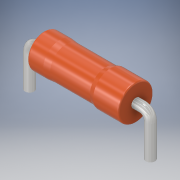
# Autodesk Inventor part: Res
Saved by Autodesk Inventor 2017 (Build 210142000, 142)
## iProperties
Created: 2016-07-07
Part Number: Res
Material: Generic
Document SubType Name: Modeling
Designer: Home
Density: 1 g/cm^3
Appearance: Default
Author: Home
Autodesk Inventor part; units mm, degrees
sketch "Sketch4" plane through (0, 0, 0) normal (0, 1, 0) x (-1, 0, 0)
  circle A0 centre (3.81, 0) radius 0.29
  circle A1 centre (-3.81, 0) radius 0.29
  point P0 (0, 0)
  dimension "d24" = 3.81
  dimension "d25" = 3.81
  dimension "d26" = 0.58
  dimension "d27" = 0.58
  constraints: 2 centre point
  measures "d24" distance of point (0, 0) A0.centre
  measures "d25" distance of A1.centre point (0, 0)
  measures "d26" diameter of A0
  measures "d27" diameter of A1
extrude "Extrusion2" add sketch "Sketch4" along normal blind 1.1 and the other way blind 1
sketch "Cable-Outline" plane through (0, 0, 0) normal (0, 0, 1) x (1, 0, 0)
  arc A0 (-3.32, 1.88) -> (-4.1, 1.1) centre (-3.32, 1.1) ccw construction
  line L0 (-3.52, 1.1) -> (-4.1, 1.1) construction
  arc A1 (-3.32, 1.3) -> (-3.52, 1.1) centre (-3.32, 1.1) ccw construction
  line L1 (4.1, 1.1) -> (3.52, 1.1) construction
  arc A2 (3.52, 1.1) -> (3.32, 1.3) centre (3.32, 1.1) ccw construction
  arc A3 (4.1, 1.1) -> (3.32, 1.88) centre (3.32, 1.1) ccw construction
  line L2 (3.32, 1.1) -> (3.32, 1.88) construction
  line L3 (3.32, 1.1) -> (4.1, 1.1) construction
  line L4 (-3.32, 1.88) -> (3.32, 1.88) construction
  line L5 (-3.32, 1.3) -> (3.32, 1.3) construction
  line L6 (-3.4614, 1.2414) -> (-3.8715, 1.6515) construction
  line L7 (3.8715, 1.6515) -> (3.4614, 1.2414) construction
  line L8 (-3.6665, 1.4465) -> (-3.8476, 1.2654) construction
  line L9 (3.6665, 1.4465) -> (3.813, 1.3) construction
  point P0 (0, 0)
  point P1 (0, 1.88)
  point P2 (0, 1.3)
  dimension "d33" = 0.2
  dimension "d36" = 90
  dimension "d37" = 90
  dimension "d38" = 0.58
  dimension "d39" = 90
  dimension "d40" = 90
  dimension "d41" = 0.2
  dimension "d42" = 0.58
  dimension "d43" = 3.32
  dimension "d46" = 90
  dimension "d47" = 90
  constraints: 16 end point, 13 point on circle, 4 centre point, 4 midpoint, 2 coincident, 1 parallel
  measures "d33" radius of A1
  measures "d38" radial gap between concentric circles of A0 A1
  measures "d39" angle of L3 L2
  measures "d41" distance of A2.centre A2.end
  measures "d42" radial gap between concentric circles of A3 A2
  measures "d43" distance of point (0, 1.88) L2.end
  measures "d46" angle of L6 L8
  measures "d47" angle of L7 L9
sketch "Cable-Center" plane through (0, 0, 0) normal (1, 0, 0) x (0, 1, 0)
  line L0 (1.3, 0) -> (1.88, 0) construction
  circle A0 centre (1.59, 0) radius 0.29
  point P0 (0, 0)
  dimension "d82" = 0.58
  constraints: 2 end point, 1 centre point, 1 horizontal, 1 midpoint
  measures "d82" diameter of A0
extrude "Extrusion3" add sketch "Cable-Center" along normal mid plane 6.64
ref_plane "Cable-Plane-A" through (-3.6665, 1.4465, 0) normal (-0.7071068, -0.7071068, 0) x (0.7071068, -0.7071068, 0)
sketch "Cable-Sketch-A" plane through (-3.6665, 1.4465, 0) normal (-0.7071068, -0.7071068, 0) x (0.7071068, -0.7071068, 0)
  circle A0 centre (0, 0) radius 0.29
  point P0 (3.6154, 0)
  dimension "d50" = 0.58
  constraints: 1 centre point
  measures "d50" diameter of A0
ref_plane "Cable-Plane-B" through (3.6665, 1.4465, 0) normal (0.7071068, -0.7071068, 0) x (0.7071068, 0.7071068, 0)
sketch "Cable-Sketch-B" plane through (3.6665, 1.4465, 0) normal (0.7071068, -0.7071068, 0) x (0.7071068, 0.7071068, 0)
  circle A0 centre (0, 0) radius 0.29
  point P0 (-3.6154, 0)
  point P1 (0.29, 0)
  dimension "d81" = 0.58
  constraints: 1 centre point, 1 coincident
  measures "d81" diameter of A0
loft "Loft4" add profiles "Cable-Sketch-B" section 1 edges at (4.1, 1.1, 0) section 3 edges at (3.32, 1.3, 0)
loft "Loft5" add profiles "Cable-Sketch-A" section 1 edges at (-3.52, 1.1, 0) section 3 edges at (-3.32, 1.3, 0)
ref_plane "Coat-Plane" through (0, 1.59, 0) normal (0, 1, 0) x (-1, 0, 0)
sketch "Coat-Cut" plane through (0, 1.59, 0) normal (0, 1, 0) x (-1, 0, 0)
  line L0 (3.32, -0.29) -> (-3.32, -0.29) projected
  line L1 (2.9, 0.29) -> (-2.9, 0.29)
  line L2 (-2.9, 0.29) -> (-2.9, -0.29)
  line L3 (-2.9, -0.29) -> (2.9, -0.29)
  line L4 (2.9, -0.29) -> (2.9, 0.29)
  line L5 (2.9, 0.29) -> (-2.9, -0.29) construction
  line L6 (-2.9, 0.29) -> (2.9, -0.29) construction
  point P0 (0, 0)
  dimension "d63" = 5.8
  constraints: 12 end point, 2 midpoint, 2 parallel, 1 horizontal, 1 perpendicular, 1 point on line
  measures "d63" distance of L3.end L2.end
sketch "Sketch11" plane through (0, 1.59, 0) normal (0, 1, 0) x (-1, 0, 0)
  circle A0 centre (3.81, 0) radius 0.29 projected
  line L0 (4.1, 0) -> (-4.1, 0)
  circle A1 centre (-3.81, 0) radius 0.29 projected
  line L1 (2.8998, -0.29) -> (2.8998, -0.95)
  line L2 (-1.0003, -1.01) -> (-1.3002, -1.1)
  line L3 (-1.3002, -1.1) -> (-2.8002, -1.1)
  line L4 (-2.9002, -1) -> (-2.9002, -0.29)
  arc A2 (-2.9002, -1) -> (-2.8002, -1.1) centre (-2.8002, -1) ccw
  line L5 (2.8998, -0.29) -> (-2.9002, -0.29)
  line L6 (3.32, -0.29) -> (-3.32, -0.29) projected
  line L7 (2.7998, -1.05) -> (1.8998, -1.05)
  line L8 (1.8998, -1.05) -> (1.4997, -1.01)
  line L9 (1.4997, -1.01) -> (-1.0003, -1.01)
  arc A3 (2.7998, -1.05) -> (2.8998, -0.95) centre (2.7998, -0.95) ccw
  point P0 (0, 0)
  point P1 (0, 0)
  point P2 (-2.9002, -1.1)
  point P3 (2.8998, -1.05)
  point P4 (-0.0002, -0.29)
  dimension "d67" = 0.81
  dimension "d68" = 1.6
  dimension "d69" = 0.1
  dimension "d72" = 0.76
  dimension "d73" = 1
  dimension "d74" = 2.5
  dimension "d75" = 0.1
  dimension "d76" = 0.72
  dimension "d83" = 0.29
  constraints: 18 end point, 5 point on line, 4 point on circle, 4 tangent, 3 parallel, 2 centre point, 2 horizontal, 2 horizontal alignment, 2 midpoint, 1 coincident, 1 collinear, 1 vertical, 2 other
  measures "d67" distance of point (-2.9, -1.1) L4.end
  measures "d68" distance of L2.end point (-2.9, -1.1)
  measures "d69" radius of A2
  measures "d72" distance of L1.start point (2.9, -1.05)
  measures "d73" distance of point (2.9, -1.05) L7.end
  measures "d74" distance of L8.end L2.start
  measures "d75" radius of A3
  measures "d76" distance between parallel lines of L5 L9
  measures "d83" distance of point (0, 0) point (0, -0.29)
revolve "Coat-Body" add sketch "Sketch11" angle 360 about axis through (-4.1, 1.59, 0) along (1, 0, 0) separate body contours L1 A3 L7 L8 L9 L2 L3 A2 L4 L5
equation "\"d27\" = d26"
equation "\"d82\" = d26"
equation "\"d44\" = 2 * d43"
equation "\"d50\" = d26"
equation "\"d81\" = d26"
equation "\"d83\" = 0.5 * d26"
